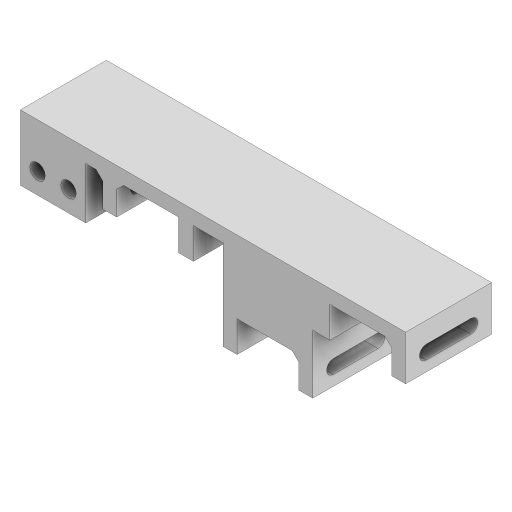
# Autodesk Inventor part: adapter_ver.1
Saved by Autodesk Inventor 2024 (Build 280153000, 153)
## iProperties
Created: 2023-11-09
Part Number: adapter_ver.1
Material: 一般
Document SubType Name: Modeling
Designer: moonshot
Density: 1 g/cm^3
Appearance: 既定
Author: moonshot
Autodesk Inventor part; units mm, degrees
ref_plane "YZ Plane" through (0, 0, 0) normal (1, 0, 0) x (0, 1, 0)
sketch "スケッチ1" plane through (0, 0, 0) normal (0, 0, 1) x (1, 0, 0)
  line L0 (94.5, 10.9383) -> (94.5, -2.0617)
  line L1 (67.5, -2.0617) -> (67.5, -19.1729)
  line L2 (45.5, -19.1729) -> (45.5, -10.1729)
  line L3 (45.5, -10.1729) -> (63.5, -10.1729)
  line L4 (63.5, -10.1729) -> (63.5, -19.1729)
  line L5 (67.5, -19.1729) -> (63.5, -19.1729)
  line L6 (45.5, -19.1729) -> (41.5, -19.1729)
  line L7 (72.5, -2.0617) -> (72.5, 6.9383)
  line L8 (72.5, 6.9383) -> (90.5, 6.9383)
  line L9 (90.5, 6.9383) -> (90.5, -2.0617)
  line L10 (45.5, -19.1729) -> (55.5, -19.1729) construction
  line L11 (55.5, -19.1729) -> (55.5, -10.1729) construction
  line L12 (50.5, -19.1729) -> (50.5, 17.1682) construction
  line L13 (28.5, -2.0617) -> (28.5, 6.9383)
  line L14 (28.5, 6.9383) -> (10.5, 6.9383)
  line L15 (10.5, 6.9383) -> (10.5, -2.0617)
  line L16 (-17.5, 10.9383) -> (94.5, 10.9383)
  line L17 (94.5, -2.0617) -> (90.5, -2.0617)
  line L18 (72.5, -2.0617) -> (67.5, -2.0617)
  line L19 (6.5, -2.0617) -> (10.5, -2.0617)
  line L20 (6.5, -2.0617) -> (6.5, 6.9383)
  line L21 (6.5, 6.9383) -> (1.5, 6.9383)
  line L22 (72.5, -2.0617) -> (82.5, -2.0617) construction
  line L23 (82.5, -2.0617) -> (82.5, 6.9383) construction
  line L24 (77.5, -2.0617) -> (77.5, 30.8698) construction
  line L25 (28.5, -2.0617) -> (18.5, -2.0617) construction
  line L26 (18.5, -2.0617) -> (18.5, 6.9383) construction
  line L27 (23.5, -2.0617) -> (23.5, 26.9166) construction
  line L28 (41.5, -19.1729) -> (41.5, 6.9383)
  line L29 (41.5, 6.9383) -> (32.8043, 6.9383)
  line L30 (32.8043, 6.9383) -> (32.8043, -2.0617)
  line L31 (32.8043, -2.0617) -> (28.5, -2.0617)
  line L32 (68.5, 6.9383) -> (45.5, 6.9383)
  line L33 (45.5, 6.9383) -> (45.5, -6.1729)
  line L34 (45.5, -6.1729) -> (60.5869, -6.1729)
  line L35 (60.5869, -6.1729) -> (68.5, 1.7403)
  line L36 (68.5, 1.7403) -> (68.5, 6.9383)
  line L37 (0, -29.1814) -> (0, 40.8784) projected
  line L38 (1.5, 6.9383) -> (1.5, -8.0617)
  line L39 (1.5, -8.0617) -> (-17.5, -8.0617)
  line L40 (-17.5, -8.0617) -> (-17.5, 10.9383)
  circle A0 centre (-12.5, -2.0617) radius 2.25
  circle A1 centre (-3.5, -2.0617) radius 2.25
  line L41 (-12.5, -2.0617) -> (-3.5, -2.0617) construction
  point P0 (0, 0)
  point P1 (68.5, 4.3393)
  point P2 (68.5, 4.4383)
  dimension "d5" = 4
  dimension "d10" = 18
  dimension "d14" = 18
  dimension "d16" = 10
  dimension "d19" = 9
  dimension "d23" = 4
  dimension "d40" = 4
  dimension "d41" = 9
  dimension "d42" = 10
  dimension "d43" = 10
  dimension "d74" = 4
  dimension "d89" = 4
  dimension "d90" = 135
  dimension "d91" = 4
  dimension "d92" = 4
  dimension "d93" = 4
  dimension "d94" = 4
  dimension "d104" = 5
  dimension "d105" = 19
  dimension "d107" = 4.5
  dimension "d108" = 4.5
  dimension "d109" = 9
  dimension "d110" = 5
  dimension "d111" = 6
  dimension "d112" = 19
  constraints: 82 end point, 26 perpendicular, 4 horizontal, 4 midpoint, 4 symmetric about line, 4 vertical, 3 collinear, 3 point on line, 2 centre point, 1 parallel, 1 other
  measures "d5" distance of L2.start L6.end
  measures "d10" distance of L2.end L3.end
  measures "d14" distance of L7.end L8.end
  measures "d16" distance of L2.start L10.end
  measures "d19" distance of L2.start L2.end
  measures "d23" distance between parallel lines of L0 L9
  measures "d40" distance of L19.start L15.end
  measures "d41" distance of L7.start L7.end
  measures "d42" distance of L7.start L22.end
  measures "d43" distance of L13.start L25.end
  measures "d74" distance between parallel lines of L21 L16
  measures "d89" distance of L1.end L4.end
  measures "d90" angle of L35 L34
  measures "d91" distance from line of point (68.5, 4.339) L7
  measures "d92" distance between parallel lines of L16 L32
  measures "d93" distance between parallel lines of L28 L33
  measures "d94" distance between parallel lines of L3 L34
  measures "d104" distance between parallel lines of L20 L38
  measures "d105" distance of L38.end L39.end
  measures "d107" diameter of A0
  measures "d108" diameter of A1
  measures "d109" distance of L41.end L41.start
  measures "d110" distance from line of L40 L41.start
  measures "d111" distance from line of L41.start L39
  measures "d112" distance of L39.end L16.start
extrude "押し出し1" add sketch "スケッチ1" along normal mid plane 25 contours L0 L17 L9 L8 L7 L18 L1 L5 L4 L3 L2 L6 L28 L29 L30 L31 L13 L14 L15 L19 L20 L21 L38 L39 L37 L16 | L37 L39 L40 L16 | L36 L35 L34 L33 L32
sketch "スケッチ2" plane through (67.5, -19.1729, 12.5) normal (1, 0, 0) x (0, 0, -1)
  line L0 (6, 3) -> (19, 3)
  arc A0 (19, 3) -> (19, 7) centre (19, 5) ccw
  line L1 (19, 7) -> (6, 7)
  arc A1 (6, 7) -> (6, 3) centre (6, 5) ccw
  line L2 (25, 0) -> (0, 0) projected
  line L3 (25, 17.1112) -> (25, 0) projected
  line L4 (0, 0) -> (0, 17.1112) projected
  point P0 (12.5, 19.1729)
  point P1 (25, 13)
  point P2 (0, 13)
  dimension "d24" = 4
  dimension "d25" = 3
  dimension "d26" = 6
  dimension "d27" = 6
  constraints: 4 end point, 4 point on circle, 4 tangent, 2 centre point, 1 horizontal, 1 parallel
  measures "d24" distance between parallel lines of L0 L1
  measures "d25" distance between parallel lines of L2 L0
  measures "d26" distance from line of L3 A0.centre
  measures "d27" distance from line of L4 A1.centre
extrude "押し出し2" cut sketch "スケッチ2" against normal up to surface (4 mm away)
chamfer "面取り1" distance 2 angle 45 1 edges at (63.5, -10.1729, 0)
sketch "スケッチ4" plane through (94.5, -2.0617, 12.5) normal (1, 0, 0) x (0, 0, -1)
  line L0 (6, 3) -> (19, 3)
  arc A0 (19, 3) -> (19, 7) centre (19, 5) ccw
  line L1 (19, 7) -> (6, 7)
  arc A1 (6, 7) -> (6, 3) centre (6, 5) ccw
  line L2 (25, 13) -> (25, 0) projected
  line L3 (0, 0) -> (0, 13) projected
  line L4 (25, 0) -> (0, 0) projected
  point P0 (12.5, 2.0617)
  dimension "d45" = 4
  dimension "d46" = 6
  dimension "d47" = 6
  dimension "d48" = 3
  constraints: 4 end point, 4 point on circle, 4 tangent, 2 centre point, 2 horizontal
  measures "d45" distance between parallel lines of L0 L1
  measures "d46" distance from line of L2 A0.centre
  measures "d47" distance from line of L3 A1.centre
  measures "d48" distance between parallel lines of L4 L0
extrude "押し出し3" cut sketch "スケッチ4" against normal up to surface (4 mm away)
sketch "スケッチ5" plane through (6.5, -2.0617, 12.5) normal (-1, 0, 0) x (0, 0, 1)
  line L0 (-19, 3) -> (-6, 3) projected
  line L1 (-19, 3) -> (-6, 3)
  arc A0 (-6, 3) -> (-6, 7) centre (-6, 5) ccw
  line L2 (-6, 7) -> (-19, 7) projected
  line L3 (-6, 7) -> (-19, 7)
  arc A1 (-19, 7) -> (-19, 3) centre (-19, 5) ccw
  point P0 (-12.5, 2.0617)
  point P1 (-6, 7)
  constraints: 4 end point, 4 point on circle, 4 tangent, 2 centre point, 2 equal length
extrude "押し出し4" cut sketch "スケッチ5" against normal up to surface (4 mm away)
chamfer "面取り4" distance 2 angle 45 3 edges at (90.5, 6.9383, 0) (10.5, 6.9383, 0) (6.5, 6.9383, 0)
ref_plane "作業平面1" through (0, 0, 1.5) normal (0, 0, 1) x (1, 0, 0)
ref_plane "作業平面2" through (0, 0, 0.1) normal (0, 0, 1) x (1, 0, 0)
